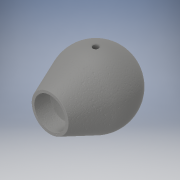
# Autodesk Inventor part: FilmLamp
Saved by Autodesk Inventor 2018.2 (Build 222227000, 227)
## iProperties
Created: 2018-01-26
Part Number: FilmLamp
Material: Beton
Document SubType Name: Modeling
Designer: JochenAlt
Density: 2.40731 g/cm^3
Appearance: Textur - grau
Mass: 1335.7 g
Surface Area: 867.6 cm^2
Volume: 554.85 cm^3
Author: JochenAlt
Autodesk Inventor part; units mm, degrees
ref_plane "YZ Plane" through (0, 0, 0) normal (1, 0, 0) x (0, 1, 0)
ref_plane "XZ Plane" through (0, 0, 0) normal (0, 1, 0) x (-1, 0, 0)
ref_plane "XY Plane" through (0, 0, 0) normal (0, 0, 1) x (1, 0, 0)
sketch "Skizze1" plane through (0, 0, 0) normal (0, 0, 1) x (1, 0, 0)
  line L0 (0, 104.266) -> (0, -111.9697) construction
  line L1 (-21.501, 0) -> (94.0062, 0) construction
  line L2 (6, 60.7042) -> (6, 37.6387)
  line L3 (25.2446, -55.1591) -> (27.5, -80.9387)
  line L4 (31.8318, -80.9387) -> (27.5, -80.9387)
  arc A0 (56.3567, -23.3437) -> (6, 60.7042) centre (0, 0) ccw
  line L5 (56.3567, -23.3437) -> (32.7557, -80.3214)
  arc A1 (31.8318, -80.9387) -> (32.7557, -80.3214) centre (31.8318, -79.9387) ccw
  circle A2 centre (0, 0) radius 5
  arc A3 (25.2446, -55.1591) -> (6, 37.6387) centre (0, -12) ccw
  line L6 (52.114, -33.5863) -> (46.194, -31.1342) construction
  point P0 (32.5, -80.9387)
  dimension "d3" = 6
  dimension "d12" = 5
  dimension "d15" = 5
  dimension "d16" = 27.5
  dimension "d17" = 1
  dimension "d18" = 10
  dimension "d68" = 100
  dimension "d69" = 12
  dimension "d71" = 25.7796
  dimension "d72" = 23.0655
  dimension "d73" = 22.5
  dimension "d76" = 61
  dimension "d77" = 6.4078
  constraints: 10 end point, 7 point on circle, 4 centre point, 4 point on line, 3 tangent, 2 coincident, 1 horizontal, 1 line through centre, 1 perpendicular, 1 vertical
  measures "d3" distance between parallel lines of L2 L0
  measures "d12" angle of L0 L3
  measures "d15" distance of point (32.5, -80.939) L3.end
  measures "d16" distance from line of L0 L3.end
  measures "d17" radius of A1
  measures "d18" diameter of A2
  measures "d68" diameter of A3
  measures "d69" distance of A3.centre point (0, 0)
  measures "d71" vertical distance of L3.start L3.end
  measures "d72" distance of L2.start L2.end
  measures "d73" angle of L0 L5
  measures "d76" radius of A0
  measures "d77" distance of L6.start L6.end
revolve "Umdrehung1" add sketch "Skizze1" angle 360 about axis through (0, 0, 0) along (0, -1, 0) contours A0 L5 A1 L4 L3 A3 L2
extrude "Extrusion1" cut sketch "Skizze1" along normal through all both and the other way through all contours A2
sketch "Skizze3" plane through (0, 0, 0) normal (0, 0, 1) x (1, 0, 0)
  point P0 (0, 0)
